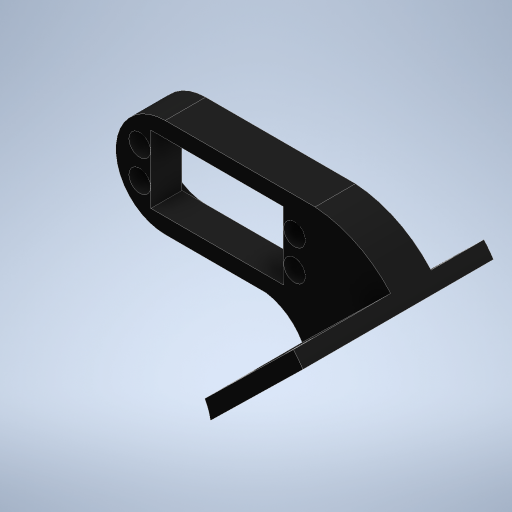
# Autodesk Inventor part: Ramie1
Saved by Autodesk Inventor 2024.2 (Build 282272000, 272)
## iProperties
Created: 2023-11-11
Part Number: Ramie1
Material: Ogólny
Document SubType Name: Modeling
Designer: nosal
Density: 1 g/cm^3
Appearance: Domyślna
Author: nosal
## iProperties of the stored document Ramie1_Drukowanie 3D.ipt
Created: 2023-11-12
Part Number: Ramie1_Drukowanie 3D
Material: Ogólny
Document SubType Name: Modeling
Designer: nosal
Density: 1 g/cm^3
Appearance: Domyślna
Author: nosal
Autodesk Inventor part; units mm, degrees
ref_plane "YZ Plane" through (0, 0, 0) normal (1, 0, 0) x (0, 1, 0)
ref_plane "XZ Plane" through (0, 0, 0) normal (0, 1, 0) x (-1, 0, 0)
ref_plane "XY Plane" through (0, 0, 0) normal (0, 0, 1) x (1, 0, 0)
sketch "Szkic1" plane through (0, 0, 0) normal (0, 0, 1) x (1, 0, 0)
  line L0 (20.3, -9.9) -> (-20.3, -9.9)
  line L1 (-20.3, -9.9) -> (-20.3, 9.9)
  line L2 (-20.3, 9.9) -> (20.3, 9.9)
  line L3 (20.3, 9.9) -> (20.3, -9.9)
  line L4 (20.3, -9.9) -> (-20.3, 9.9) construction
  line L5 (-20.3, -9.9) -> (20.3, 9.9) construction
  line L6 (21.3, 10.9) -> (-21.3, 10.9)
  line L7 (-21.3, 10.9) -> (-21.3, -10.9)
  line L8 (-21.3, -10.9) -> (21.3, -10.9)
  line L9 (21.3, -10.9) -> (21.3, 10.9)
  line L10 (0, 0) -> (24.89, 0)
  line L11 (24.89, 0) -> (24.89, 5)
  line L12 (24.89, 5) -> (24.89, -5)
  line L13 (0, 0) -> (-24.89, 0)
  line L14 (-24.89, 5) -> (-24.89, 0)
  line L15 (-24.89, 0) -> (-24.89, -5)
  circle A0 centre (-24.89, 5) radius 1.621
  circle A1 centre (-24.89, -5) radius 1.621
  circle A2 centre (24.89, -5) radius 1.621
  circle A3 centre (24.89, 5) radius 1.621
  line L16 (-26.511, 5) -> (-31.511, 5)
  line L17 (26.511, 5) -> (31.511, 5)
  line L18 (0, 10.9) -> (0, 15.9)
  line L19 (0, 15.9) -> (-16.6819, 15.9)
  line L20 (0, -10.9) -> (0, -15.9)
  line L21 (0, -15.9) -> (-16.6819, -15.9)
  line L22 (-31.511, -5.7364) -> (-31.511, 5.7364)
  line L23 (0, 15.9) -> (31.511, 15.9)
  line L24 (31.511, 15.9) -> (31.511, -15.9)
  line L25 (0, -15.9) -> (31.511, -15.9)
  arc A4 (58.9078, 0) -> (31.511, 15.9) centre (29.1703, -19.6864) ccw
  arc A5 (29.1703, -29.1056) -> (15.7555, -15.9) centre (13.2559, -31.8556) ccw
  line L26 (29.1703, -29.1056) -> (58.9078, 0)
  circle A6 centre (-16.6819, 0) radius 15.9
  arc A7 (-32.5353, -15.867) -> (-31.511, -15.9) centre (-31.511, 0) ccw
  point P0 (58.9078, 0)
  dimension "d10" = 3.242
  dimension "d13" = 3.242
  dimension "d0" = 40.6
  dimension "d1" = 19.8
  dimension "d2" = 1
  dimension "d3" = 42.6
  dimension "d4" = 24.89
  dimension "d5" = 5
  dimension "d6" = 10
  dimension "d7" = 24.89
  dimension "d8" = 5
  dimension "d9" = 5
  dimension "d11" = 3.242
  dimension "d12" = 3.242
  dimension "d14" = 5
  dimension "d15" = 5
  dimension "d16" = 5
  dimension "d17" = 5
  dimension "d18" = 6.621
  dimension "d19" = 63.022
  dimension "d20" = 10.9
  dimension "d21" = 0
  constraints: 54 end point, 11 point on circle, 8 perpendicular, 6 centre point, 6 horizontal, 6 midpoint, 5 point on line, 4 coincident, 4 parallel, 3 vertical, 2 horizontal alignment, 1 tangent, 7 other
  measures "d0" distance of L1.end L2.end
  measures "d1" distance of L0.end L1.end
  measures "d2" distance between parallel lines of L2 L6
  measures "d3" distance of L6.start L6.end
  measures "d4" distance of L10.start L10.end
  measures "d5" distance of L10.end L11.end
  measures "d6" distance of L11.end L12.end
  measures "d7" distance of L10.start L13.end
  measures "d8" distance of L14.start L13.end
  measures "d9" distance of L13.end L15.end
  measures "d11" diameter of A1
  measures "d12" diameter of A2
  measures "d14" distance of L16.start L16.end
  measures "d15" distance of L17.start L17.end
  measures "d16" distance of L18.start L18.end
  measures "d17" distance of L20.start L20.end
  measures "d18" distance between parallel lines of L11 L24
  measures "d19" distance between parallel lines of L24 L22
  measures "d20" distance between parallel lines of L17 L23
  measures "d21" distance between parallel lines of L17 L16
extrude "Wyciągnięcie proste1" add sketch "Szkic1" along normal blind 10 contours A6 L22 L16 A0 L14 L13 L7 L8 | L8 L20 L21 A6 | L10 L11 A3 L17 L24 L25 L20 L8 L9 | L9 L6 L18 L23 L24 L17 A3 L11 L10 | L13 L14 A0 L16 L22 A6 L6 L7 | A6 L22 | A6 L19 L18 L6 | L25 L24 A4 L26 A5
sketch "Szkic2" plane through (0, 0, 10) normal (0, 0, 1) x (1, 0, 0)
  arc A0 (29.1703, -29.1056) -> (15.7555, -15.9) centre (13.2559, -31.8556) ccw projected
  line L0 (29.1703, -29.1056) -> (58.9078, 0) projected
  arc A1 (58.9078, 0) -> (31.511, 15.9) centre (29.1703, -19.6864) ccw projected
  line L1 (29.1703, -29.1056) -> (58.9078, 0) projected
  arc A2 (29.1703, -29.1056) -> (15.7555, -15.9) centre (13.2559, -31.8556) ccw projected
  line L2 (27.3214, -23.9188) -> (55.8385, 3.9923)
  line L3 (31.511, 15.9) -> (-16.6819, 15.9) projected
  arc A3 (-16.6819, 15.9) -> (-16.6819, -15.9) centre (-16.6819, 0) ccw projected
  line L4 (-16.6819, -15.9) -> (15.7555, -15.9) projected
  point P0 (0, 0)
  dimension "d24" = 5
  constraints: 2 end point, 2 point on circle, 1 parallel
  measures "d24" distance between parallel lines of L0 L2
extrude "Wyciągnięcie proste2" add sketch "Szkic2" along normal blind 20 contours A0 L2 A1 L0
sketch "Szkic3" plane through (0, 0, 0) normal (0, 0, -1) x (-1, 0, 0)
  line L0 (-27.3214, -23.9188) -> (-55.8385, 3.9923) projected
  line L1 (-29.1703, -29.1056) -> (-58.9078, 0) projected
  arc A0 (-15.7555, -15.9) -> (-29.1703, -29.1056) centre (-13.2559, -31.8556) ccw projected
  arc A1 (-31.511, 15.9) -> (-58.9078, 0) centre (-29.1703, -19.6864) ccw projected
  line L2 (-29.1703, -29.1056) -> (-58.9078, 0) projected
  line L3 (16.6819, -15.9) -> (-15.7555, -15.9) projected
  arc A2 (16.6819, -15.9) -> (16.6819, 15.9) centre (16.6819, 0) ccw projected
  line L4 (-31.511, 15.9) -> (16.6819, 15.9) projected
  point P0 (0, 0)
  point P1 (-55.8385, 3.9923)
extrude "Wyciągnięcie proste3" add sketch "Szkic3" along normal blind 20 contours A0 L1 A1 L0
sketch "Szkic9" plane through (0, 0, 30) normal (0, 0, 1) x (1, 0, 0)
  arc A0 (29.1703, -29.1056) -> (27.3214, -23.9188) centre (13.2559, -31.8556) ccw projected
  line L0 (29.1703, -29.1056) -> (58.9078, 0) projected
  arc A1 (58.9078, 0) -> (55.8385, 3.9923) centre (29.1703, -19.6864) ccw projected
  line L1 (55.8385, 3.9923) -> (27.3214, -23.9188) projected
  point P0 (0, 0)
extrude "Wyciągnięcie proste5" add sketch "Szkic9" along normal blind 11.3
sketch "Szkic10" plane through (58.9078, 0, -20) normal (0.6995, -0.7147, 0) x (0.7147, 0.6995, 0)
  line L0 (-41.6107, 0) -> (-41.6107, 61.3) projected
  line L1 (0, 0) -> (-41.6107, 0) projected
  line L2 (0, 0) -> (0, 61.3) projected
  line L3 (-41.6107, 61.3) -> (0, 61.3) projected
  point P0 (-42.099, 20)
  point P1 (-33.6107, 8)
  point P2 (-8, 8)
  point P3 (-33.6107, 53.3)
  point P4 (-8, 53.3)
  dimension "d60" = 8
  dimension "d61" = 8
  dimension "d62" = 8
  dimension "d63" = 8
  dimension "d64" = 8
  dimension "d65" = 8
  dimension "d66" = 8
  dimension "d67" = 8
  measures "d60" distance from line of L0 point (-33.611, 8)
  measures "d61" distance from line of L1 point (-33.611, 8)
  measures "d62" distance from line of L1 point (-8, 8)
  measures "d63" distance from line of L2 point (-8, 8)
  measures "d64" distance from line of L0 point (-33.611, 53.3)
  measures "d65" distance from line of L3 point (-33.611, 53.3)
  measures "d66" distance from line of L3 point (-8, 53.3)
  measures "d67" distance from line of L2 point (-8, 53.3)
hole "Otwór2" at (34.8876, -23.5098, -12) at (53.1905, -5.5958, -12) at (34.8876, -23.5098, 33.3) at (53.1905, -5.5958, 33.3) direction (-0.6995, 0.7147, 0) diameter 3.242 end through all thread size "M4x0.7" designation "M4" class "6H" standard "GB Metric profile"
sketch "Szkic12" plane through (55.8385, 3.9923, 0) normal (-0.6995, 0.7147, 0) x (0.7147, 0.6995, 0)
  circle A0 centre (-34.2097, 12) radius 1.621 projected
  circle A1 centre (-8.599, 12) radius 1.621 projected
  line L0 (0, 0) -> (-39.9031, 0) projected
  line L1 (0, 0) -> (0, 20) projected
  line L2 (-39.9031, 20) -> (0, 20) projected
  line L3 (-39.9031, 0) -> (-39.9031, 20) projected
  circle A2 centre (-34.2097, -33.3) radius 1.621 projected
  circle A3 centre (-8.599, -33.3) radius 1.621 projected
  line L4 (-39.9031, -10) -> (0, -10) projected
  line L5 (-39.9031, -10) -> (-39.9031, -41.3) projected
  line L6 (0, -41.3) -> (-39.9031, -41.3) projected
  line L7 (0, -10) -> (0, -41.3) projected
  circle A4 centre (-8.599, 12) radius 1.621 projected
  circle A5 centre (-8.599, 12) radius 3.5
  circle A6 centre (-34.2097, 12) radius 3.5
  circle A7 centre (-34.2097, -33.3) radius 3.5
  circle A8 centre (-8.599, -33.3) radius 3.5
  point P0 (-42.698, 0)
  dimension "d77" = 7
  dimension "d78" = 7
  dimension "d79" = 7
  dimension "d80" = 7
  constraints: 4 centre point, 4 coincident
  measures "d77" diameter of A5
  measures "d78" diameter of A6
  measures "d79" diameter of A7
  measures "d80" diameter of A8
extrude "Wyciągnięcie proste6" cut sketch "Szkic12" against normal blind 3 contours A0 | A1 | A2 | A3 | A5 | A6 | A7 | A8
sketch "Szkic15" plane through (0, 0, 0) normal (0, 0, -1) x (-1, 0, 0)
  line L0 (-55.8385, 3.9923) -> (-27.3214, -23.9188) projected
  arc A0 (-15.7555, -15.9) -> (-27.3214, -23.9188) centre (-13.2559, -31.8556) ccw projected
  line L1 (16.6819, -15.9) -> (-15.7555, -15.9) projected
  arc A1 (16.6819, -15.9) -> (16.6819, 15.9) centre (16.6819, 0) ccw projected
  line L2 (-31.511, 15.9) -> (16.6819, 15.9) projected
  arc A2 (-31.511, 15.9) -> (-55.8385, 3.9923) centre (-29.1703, -19.6864) ccw projected
  circle A3 centre (24.89, 5) radius 1.621 projected
  circle A4 centre (24.89, -5) radius 1.621 projected
  line L3 (-21.3, 10.9) -> (-21.3, -10.9) projected
  line L4 (21.3, 10.9) -> (-21.3, 10.9) projected
  line L5 (21.3, -10.9) -> (21.3, 10.9) projected
  line L6 (-21.3, -10.9) -> (21.3, -10.9) projected
  circle A5 centre (-24.89, -5) radius 1.621 projected
  circle A6 centre (-24.89, 5) radius 1.621 projected
  arc A7 (16.6819, -13.9) -> (16.6819, 13.9) centre (16.6819, 0) ccw
  line L7 (16.6819, -13.9) -> (-15.9066, -13.9)
  arc A8 (-15.9066, -13.9) -> (-27.6497, -20.799) centre (-13.2559, -31.8556) ccw
  line L8 (-27.6497, -20.799) -> (-53.0395, 4.0513)
  arc A9 (-31.4443, 13.9) -> (-53.0395, 4.0513) centre (-29.1703, -19.6864) ccw
  line L9 (-31.4443, 13.9) -> (16.6819, 13.9)
  line L10 (-53.0395, 4.0513) -> (-54.4074, 2.5916)
  line L11 (-55.8385, 3.9923) -> (-27.3214, -23.9188) projected
  line L12 (-27.6497, -20.799) -> (-29.0176, -22.2587)
  point P0 (0, 0)
  dimension "d86" = 2
  constraints: 10 end point, 6 point on circle, 3 centre point, 2 point on line, 1 parallel, 5 other
  measures "d86" distance between parallel lines of L2 L9
extrude "Wyciągnięcie proste8" add sketch "Szkic15" along normal blind 3 contours A2 L2 A1 L1 A0 L0 L12 A8 L7 A7 L9 A9 L10
sketch "Szkic17" plane through (0, 0, 10) normal (0, 0, 1) x (1, 0, 0)
  line L0 (27.3214, -23.9188) -> (55.8385, 3.9923) projected
  arc A0 (55.8385, 3.9923) -> (31.511, 15.9) centre (29.1703, -19.6864) ccw projected
  line L1 (31.511, 15.9) -> (-16.6819, 15.9) projected
  arc A1 (-16.6819, 15.9) -> (-16.6819, -15.9) centre (-16.6819, 0) ccw projected
  line L2 (-16.6819, -15.9) -> (15.7555, -15.9) projected
  arc A2 (27.3214, -23.9188) -> (15.7555, -15.9) centre (13.2559, -31.8556) ccw projected
  circle A3 centre (-24.89, 5) radius 1.621 projected
  circle A4 centre (-24.89, -5) radius 1.621 projected
  line L3 (21.3, 10.9) -> (21.3, -10.9) projected
  line L4 (21.3, -10.9) -> (-21.3, -10.9) projected
  line L5 (-21.3, -10.9) -> (-21.3, 10.9) projected
  line L6 (-21.3, 10.9) -> (21.3, 10.9) projected
  circle A5 centre (24.89, -5) radius 1.621 projected
  circle A6 centre (24.89, 5) radius 1.621 projected
  circle A7 centre (-24.89, -5) radius 3.5
  circle A8 centre (-24.89, 5) radius 1.621 projected
  circle A9 centre (-24.89, 5) radius 3.5
  circle A10 centre (24.89, -5) radius 3.5
  circle A11 centre (24.89, 5) radius 3.5
  point P0 (0, 0)
  dimension "d89" = 7
  dimension "d90" = 7
  dimension "d91" = 7
  dimension "d92" = 7
  constraints: 4 centre point, 4 coincident
  measures "d89" diameter of A7
  measures "d90" diameter of A9
  measures "d91" diameter of A10
  measures "d92" diameter of A11
extrude "Wyciągnięcie proste9" cut sketch "Szkic17" against normal blind 6 contours A7 | A9 | A10 | A11
equation "\"d13\" = d10"
equation "\"d11\" = d10"
equation "\"d12\" = d10"
equation "\"d62\" = d61"
equation "\"d63\" = d62"
